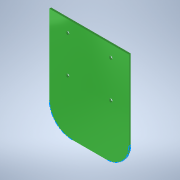
# Autodesk Inventor part: PCB-Bottom
Saved by Autodesk Inventor 2022 (Build 260153000, 153)
## iProperties
Created: 2024-05-30
Part Number: PCB-Bottom
Material: 一般
Document SubType Name: Modeling
Designer: yamashita1
Density: 1 g/cm^3
Appearance: 滑らか - 濃い深緑
Author: yamashita1
Autodesk Inventor part; units mm, degrees
ref_plane "YZ Plane" through (0, 0, 0) normal (1, 0, 0) x (0, 1, 0)
ref_plane "XZ Plane" through (0, 0, 0) normal (0, 1, 0) x (-1, 0, 0)
ref_plane "XY Plane" through (0, 0, 0) normal (0, 0, 1) x (1, 0, 0)
sketch "スケッチ1" plane through (0, 0, 0) normal (0, 0, 1) x (1, 0, 0)
  line L0 (-35, 45) -> (35, 45)
  line L1 (35, 45) -> (35, -45)
  line L2 (35, -45) -> (-35, -45)
  line L3 (-35, -45) -> (-35, 45)
  point P0 (0, 0)
  point P1 (0, 45)
  point P2 (-35, 0)
  dimension "d0" = 70
  dimension "d1" = 90
  constraints: 8 end point, 2 midpoint, 2 parallel, 1 horizontal, 1 horizontal alignment, 1 perpendicular, 1 vertical alignment
  measures "d0" distance of L1.end L2.end
  measures "d1" distance of L0.end L1.end
extrude "押し出し1" add sketch "スケッチ1" along normal blind 1.6
fillet "フィレット1" radius 20 2 edges at (35, -45, 0.8) (-35, -45, 0.8)
derived "FS90-Mount2.ipt"
sketch "スケッチ2" plane through (0, 0, 1.6) normal (0, 0, 1) x (1, 0, 0)
  line L0 (-63.092, 13) -> (63.092, 13) construction
  line L1 (35, 45) -> (-35, 45) construction
  line L2 (-44.3089, 1.95) -> (50.6662, 1.95) construction
  line L3 (50.6662, 34.45) -> (-45.85, 34.45) construction
  line L4 (-23, 58.4684) -> (-23, 0) construction
  line L5 (23, 0) -> (23, 58.4684) construction
  line L6 (35, -25) -> (35, 45) construction
  line L7 (-35, 45) -> (-35, -25) construction
  circle A0 centre (0, 13) radius 57.5 construction
  point P0 (0, 0)
  point P1 (-23, 34.45)
  point P2 (-23, 1.95)
  point P3 (23, 1.95)
  point P4 (23, 34.45)
  dimension "d6" = 32
  dimension "d7" = 11.05
  dimension "d8" = 21.45
  dimension "d9" = 12
  dimension "d10" = 12
  dimension "d18" = 115
  constraints: 10 end point, 8 point on line, 2 horizontal, 1 centre point, 1 coincident, 1 midpoint, 1 perpendicular, 1 vertical alignment
  measures "d6" distance between parallel lines of L0 L1
  measures "d7" distance between parallel lines of L2 L0
  measures "d8" distance between parallel lines of L3 L0
  measures "d9" distance between parallel lines of L6 L5
  measures "d10" distance between parallel lines of L7 L4
  measures "d18" diameter of A0
hole "穴1" at (-23, 34.45, 1.6) at (-23, 1.95, 1.6) at (23, 1.95, 1.6) at (23, 34.45, 1.6) direction (0, 0, -1) diameter 3.2 end through all
equation "\"d7\" = MOUNT_X1"
equation "\"d8\" = MOUNT_X2"
equation "\"d9\" = MOUNT_Y"
equation "\"d10\" = d9"
equation "\"MOUNT_X1\" = 11.05"
equation "\"MOUNT_X2\" = 21.45"
equation "\"MOUNT_Y\" = 12"
